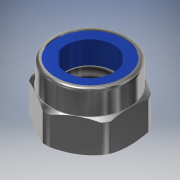
# Autodesk Inventor part: 11-4503
Saved by Autodesk Inventor 2017.1 (Build 211199000, 199)
## iProperties
Shininess: 64.0
Angle Display Precision: 2
Document Length Units: 11269
Document Angle Units: 11279
Document Time Units: 11290
Document Mass Units: 11283
Document Length Units Precision: 3
Document Angle Units Precision: 2
Compacted: True
Category: Fasteners
Company: Autodesk Inc.
Created: 2014-11-29
Part Number: 11-4503
Material: Steel, Mild
Document SubType Name: Modeling
Designer: Autodesk Inc.
Density: 7.86 g/cm^3
Appearance: Semi-Polished
Catalog Web Link: http://matrixrobotics.com/
Vendor: Matrix
Density: 0.0
Volumn: 0.0
Area: 0.0
PropertySet Name: Model Information
Control State: 0
Master: False
Checked Out: False
Author: Autodesk Inc.
Autodesk Inventor part; units mm, degrees
ref_plane "YZ Plane" through (0, 0, 0) normal (1, 0, 0) x (0, 1, 0)
ref_plane "XZ Plane" through (0, 0, 0) normal (0, 1, 0) x (-1, 0, 0)
ref_plane "XY Plane" through (0, 0, 0) normal (0, 0, 1) x (1, 0, 0)
sketch "Sketch1" plane through (0, 0, 0) normal (0, 0, 1) x (1, 0, 0)
  circle A0 centre (0, 0) radius 2
  line L0 (0, 4.0415) -> (3.5, 2.0207)
  line L1 (3.5, 2.0207) -> (3.5, -2.0207)
  line L2 (3.5, -2.0207) -> (0, -4.0415)
  line L3 (0, -4.0415) -> (-3.5, -2.0207)
  line L4 (-3.5, -2.0207) -> (-3.5, 2.0207)
  line L5 (-3.5, 2.0207) -> (0, 4.0415)
  dimension "Sw" = 7
  dimension "Diameter" = 4
  constraints: 12 end point, 1 centre point, 1 coincident, 11 other
  measures "Sw" distance between parallel lines of L0 L3
  measures "Diameter" diameter of A0
extrude "Extrusion1" add sketch "Sketch1" along normal mid plane 2.9
thread "Thread1" size "M4x0.7" class "6H" standard "ANSI Metric M Profile" length 2.9
sketch "Sketch4" plane through (0, 0, 0) normal (0, 1, 0) x (-1, 0, 0)
  line L0 (0, -1.45) -> (0, 1.45) projected
  line L1 (0, -1.45) -> (-3.5, -1.45)
  line L2 (-3.5, -1.45) -> (-4.0415, -1.1374)
  line L3 (-4.0415, -1.1374) -> (-4.0415, -1.45)
  line L4 (-4.0415, -1.45) -> (-3.5, -1.45)
  line L5 (0, -2.03) -> (0, 2.03) projected
  dimension "d6" = 4.0415
  dimension "d7" = 30
  dimension "d8" = 3.5
  constraints: 8 end point, 2 perpendicular, 1 collinear
  measures "d6" distance from line of L0.start L3
  measures "d7" angle of L2 L4
  measures "d8" distance from line of L1.end L0
revolve "Revolution1" cut sketch "Sketch4" angle 360 about axis through (0, 0, -10) along (0, 0, 1)
mirror "Mirror1" about plane through (0, 0, 0) normal (0, 0, 1) of "Revolution1"
sketch "Sketch6" plane through (0, 0, -1.45) normal (0, 0, -1) x (-1, 0, 0)
  circle A0 centre (0, 0) radius 2 projected
  circle A1 centre (0, 0) radius 3.8717
  dimension "d15" = 7.7434
  constraints: 1 centre point, 1 coincident
  measures "d15" diameter of A1
extrude "Extrusion3" cut sketch "Sketch6" against normal through all keep common part
chamfer "Chamfer2" distance 0.35 angle 45 1 edges at (-2, 0, -1.45)
sketch "Sketch8" plane through (0, 0, 1.45) normal (0, 0, 1) x (1, 0, 0)
  line L0 (-2.5, 0) -> (3.5, 0)
  circle A0 centre (0, 0) radius 3.15
  circle A1 centre (0, 0) radius 2.1
  dimension "d22" = 6.3
  dimension "d34" = 4.2
  constraints: 2 centre point, 2 coincident, 2 end point, 1 horizontal
  measures "d22" diameter of A0
  measures "d34" diameter of A1
extrude "Extrusion6" add sketch "Sketch8" along normal blind 1.995
sketch "Sketch11" plane through (0, 0, 0) normal (0, 1, 0) x (-1, 0, 0)
  line L0 (1.75, -1.45) -> (3.5, -1.45) projected
  line L1 (3.15, 3.55) -> (0, 3.55)
  line L2 (3.5, 1.45) -> (1.75, 1.45) projected
  line L3 (3.43, 3.27) -> (3.43, 1.45)
  line L4 (3.15, 1.45) -> (3.15, 3.445) projected
  line L5 (2.1, 1.45) -> (2.1, 3.445) projected
  line L6 (0, -2.4616) -> (0, 4.6196) projected
  arc A0 (3.43, 3.27) -> (3.15, 3.55) centre (3.15, 3.27) ccw
  line L7 (3.15, 3.445) -> (3.038, 3.445)
  line L8 (3.038, 3.445) -> (3.038, 3.55)
  dimension "d35" = 5
  dimension "d36" = 3.43
  dimension "d37" = 0.28
  dimension "d38" = 0.28
  dimension "d40" = 0.392
  constraints: 8 end point, 3 point on line, 2 perpendicular, 2 point on circle, 2 tangent, 1 centre point, 1 parallel, 1 vertical
  measures "d35" distance between parallel lines of L1 L0
  measures "d36" distance between parallel lines of L6 L3
  measures "d37" distance between parallel lines of L4 L3
  measures "d38" radius of A0
  measures "d40" distance between parallel lines of L8 L3
revolve "Revolution2" add sketch "Sketch11" angle 360 about axis through (0, 0, -10) along (0, 0, 1)
equation "\"d4\" = M"
equation "\"d6\" = 0.57735 * Sw"
equation "\"d8\" = 0.5 * Sw"
equation "\"d15\" = 1.10619 * Sw"
equation "\"d20\" = 0.5 * Pitch"
equation "\"d21\" = 0.5 * Pitch"
equation "\"d22\" = 0.9 * Sw"
equation "\"d34\" = 1.05 * Diameter"
equation "\"d25\" = -0.95 * M + 0.95 * h"
equation "\"d35\" = h"
equation "\"d36\" = 0.49 * Sw"
equation "\"d38\" = d37"
equation "\"d40\" = 1.4 * d38"
equation "\"M\" = 2.9"
equation "\"Pitch\" = 0.7"
equation "\"h\" = 5"
body "Solid1"
